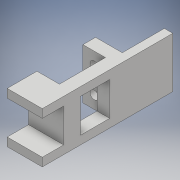
# Autodesk Inventor part: pixyCam_mount
Saved by Autodesk Inventor 2018.3 (Build 223284000, 284)
## iProperties
Created: 2020-10-16
Part Number: pixyCam_mount
Material: Generic
Document SubType Name: Modeling
Designer: chris
Density: 1 g/cm^3
Appearance: Default
Author: chris
Autodesk Inventor part; units mm, degrees
ref_plane "YZ Plane" through (0, 0, 0) normal (1, 0, 0) x (0, 1, 0)
ref_plane "XZ Plane" through (0, 0, 0) normal (0, 1, 0) x (-1, 0, 0)
ref_plane "XY Plane" through (0, 0, 0) normal (0, 0, 1) x (1, 0, 0)
sketch "Sketch1" plane through (0, 0, 0) normal (0, 0, 1) x (1, 0, 0)
  line L0 (47.7, 10.1753) -> (55.7, 10.1753)
  line L1 (55.7, -6.2247) -> (47.7, -6.2247)
  line L2 (47.7, -33.2316) -> (55.7, -33.2316)
  line L3 (55.7, -33.2316) -> (55.7, -16.8316)
  line L4 (55.7, -16.8316) -> (47.7, -16.8316)
  line L5 (60.2, -37.7316) -> (47.7, -37.7316)
  line L6 (60.2, -37.7316) -> (60.2, 14.6753)
  line L7 (55.7, -6.2247) -> (55.7, 10.1753)
  line L8 (47.7, 14.6753) -> (57.2, 14.6753)
  line L9 (47.7, -33.2316) -> (47.7, -37.7316)
  line L10 (47.7, 14.6753) -> (47.7, 10.1753)
  line L11 (47.7, -6.2247) -> (47.7, -16.8316)
  line L12 (60.2, 14.6753) -> (60.2, 29.6753)
  line L13 (60.2, 29.6753) -> (57.2, 29.6753)
  line L14 (57.2, 29.6753) -> (57.2, 14.6753)
  constraints: 30 end point, 5 perpendicular, 2 vertical, 1 horizontal, 1 parallel
extrude "Extrusion1" add sketch "Sketch1" along normal blind 18
sketch "Sketch2" plane through (0, 0, 18) normal (0, 0, 1) x (1, 0, 0)
  line L0 (60.2, 29.6753) -> (60.2, -37.7316) construction
  line L1 (47.7, -37.7316) -> (47.7, -33.2316) construction
  line L2 (60.2, -16.8316) -> (47.7, -16.8316)
  line L3 (47.7, -16.8316) -> (47.7, -37.7316)
  line L4 (47.7, -37.7316) -> (60.2, -37.7316)
  line L5 (60.2, -37.7316) -> (60.2, -16.8316)
  point P0 (0, 0)
  constraints: 8 end point, 2 parallel, 1 horizontal, 1 perpendicular, 1 point on line
extrude "Extrusion2" cut sketch "Sketch2" against normal blind 18
sketch "Sketch3" plane through (47.7, 14.6753, 0) normal (0, 1, 0) x (1, 0, 0)
  circle A0 centre (4, -4.5) radius 1.5
  circle A1 centre (4, -13.5) radius 1.5
  point P0 (-47.7, 0)
  constraints: 2 centre point
extrude "Extrusion3" cut sketch "Sketch3" against normal blind 4.5
sketch "Sketch4" plane through (47.7, -16.8316, 0) normal (-1, 0, 0) x (0, 0, 1)
  line L0 (0, 0) -> (18, 0) construction
  line L1 (15, 7.6069) -> (15, 0)
  line L2 (3, 0) -> (3, 7.6069)
  line L3 (3, 7.6069) -> (15, 7.6069)
  line L4 (3, 0) -> (15, 0)
  point P0 (0, 16.8316)
  constraints: 8 end point, 2 point on line, 1 collinear
extrude "Extrusion4" cut sketch "Sketch4" against normal blind 20
sketch "Sketch5" plane through (55.7, -6.2247, 0) normal (-1, 0, 0) x (0, 0, 1)
  line L0 (0, 0) -> (0, 16.4) construction
  line L1 (0, 0) -> (18, 0) construction
  line L2 (18, 16.4) -> (18, 0) construction
  line L3 (0, 16.4) -> (18, 16.4) construction
  line L4 (3, 13.4) -> (3, 3)
  line L5 (3, 3) -> (15, 3)
  line L6 (15, 3) -> (15, 13.4)
  line L7 (15, 13.4) -> (3, 13.4)
  point P0 (0, 6.2247)
  dimension "d17" = 3
  constraints: 8 end point, 3 other
  measures "d17" distance between parallel lines of L0 L4
extrude "Extrusion5" cut sketch "Sketch5" against normal up to next
body "Solid1"
